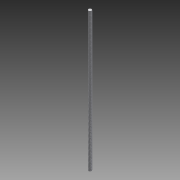
# Autodesk Inventor part: threaded rod
Saved by Autodesk Inventor 2015 (Build 190159000, 159)
## iProperties
Created: 2015-02-28
Part Number: threaded rod
Material: Generic
Document SubType Name: Modeling
Designer: Qiuyang
Density: 1 g/cm^3
Appearance: Default
Author: Qiuyang
Autodesk Inventor part; units mm, degrees
ref_plane "YZ Plane" through (0, 0, 0) normal (1, 0, 0) x (0, 1, 0)
ref_plane "XZ Plane" through (0, 0, 0) normal (0, 1, 0) x (-1, 0, 0)
ref_plane "XY Plane" through (0, 0, 0) normal (0, 0, 1) x (1, 0, 0)
sketch "Sketch1" plane through (0, 0, 0) normal (0, 1, 0) x (-1, 0, 0)
  circle A0 centre (0, 0) radius 2.413
  dimension "d0" = 4.826
  constraints: 1 centre point, 1 coincident
  measures "d0" diameter of A0
extrude "Extrusion1" add sketch "Sketch1" along normal blind 215.9
body "Solid1"
